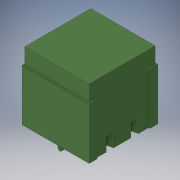
# Autodesk Inventor part: M211LW01-body
Saved by Autodesk Inventor 2019 (Build 230136000, 136)
## iProperties
Created: 2022-08-22
Part Number: M211LW01-body
Material: Generic
Catalog Web Link: www.cadenas.de
Description: Series M2100 - LED Tipped Actuators - body-
Vendor: NKKSWITCHES
Document SubType Name: Modeling
Designer: psAdmin
Manufacturer: NKKSWITCHES
Mass: 2.03481 g
Surface Area: 10.5273 cm^2
Volume: 2.03481 cm^3
Density: 1 g/cm^3
Appearance: PSOLRGB-79-119-66
Category: PARTsolutions
Company: NKKSWITCHES
Title: M211LW01-body
Author: Cadenas PARTsolutions
PSOL_IDENT_0: {$CADENAS_DATA/23d-libs/nkkswitches/toggle/m2100/parts/m2100_body.prj},219 {VTYP=3D},{NB=M211LW01-bo
PSOL_IDENT_1: dy},{LINA=M211LW01-body},{NN=Series M2100 - LED Tipped Actuators - body},{DATE=02.08.2022 07:27:12},
PSOL_IDENT_2: {GEOMDATE=10.04.2009 08:21:00},{VERSION=},{LINEID=10},{WBVAR=PLS,LCAT,CMRT,TMT},{WBNUMERIC=}  {NB=M2
PSOL_IDENT_3: 11LW01-body},{LINA=M211LW01-body},{KT=DUMMY},{PN=M211LW01},{SRS=M21},{PLS=1},{LCAT=L},{LCAT1= 'L','L
PSOL_IDENT_4: - Isolated (Toggle)','T','T - Synchronous (Toggle)','R','R - Isolated (Rocker)','N','N - Synchronou
PSOL_IDENT_5: s (Rocker)','P','P - Isolated (Paddle)','J','J - Synchronous (Paddle)' },{CMRT=W},{TMT=01},{TMT1= '0
PSOL_IDENT_6: 1','01 - Solder Lug with Threaded Bushing','02','02 - Quick Connect with Threaded Bushing','03','03
PSOL_IDENT_7: - Straight PC with Threaded Bushing' }
NB: M211LW01-body
NN: Series M2100 - LED Tipped Actuators - body
NBSYN: $PN.-body
LINA: M211LW01-body
CATALOG: NKK Switches
PN: M211LW01
SRS: M21
PLS: 1 - SPDT
LCAT: L - Isolated (Toggle)
CMRT: W - Silver; Rated 6A @ 125V AC
TMT: 01 - Solder Lug with Threaded Bushing
SUPPLIER: NKKSWITCHES
ARTICLENO: M211LW01-body
BOMINFO: M211LW01-body
CREATOR: CADENAS GmbH
Autodesk Inventor part; units mm, degrees
sketch "Sketch_1" plane through (0, 0, 0) normal (1, 0, 0) x (0, 1, 0)
  line L0 (12.8016, 6.5024) -> (0, 6.5024)
  line L1 (0, 6.5024) -> (0, -6.5024)
  line L2 (0, -6.5024) -> (12.8016, -6.5024)
  line L3 (12.8016, -6.5024) -> (12.8016, 6.5024)
  constraints: 8 end point
extrude "Extrusion1" add sketch "Sketch_1" along normal mid plane 12.7
sketch "Sketch_5" plane through (6.35, 0, 0) normal (1, 0, 0) x (0, 0, -1)
  line L0 (-6.5024, 9.7536) -> (-5.4864, 9.7536)
  arc A0 (-4.9784, 9.2456) -> (-5.4864, 9.7536) centre (-5.4864, 9.2456) ccw
  line L1 (-4.9784, 9.2456) -> (-4.9784, 0)
  line L2 (-4.9784, 0) -> (4.9784, 0)
  line L3 (4.9784, 0) -> (4.9784, 9.2456)
  arc A1 (5.4864, 9.7536) -> (4.9784, 9.2456) centre (5.4864, 9.2456) ccw
  line L4 (5.4864, 9.7536) -> (6.5024, 9.7536)
  line L5 (6.5024, 9.7536) -> (6.5024, 13.0556)
  line L6 (6.5024, 13.0556) -> (-6.5024, 13.0556)
  line L7 (-6.5024, 13.0556) -> (-6.5024, 9.7536)
  constraints: 16 end point, 4 point on circle, 2 centre point
extrude "Extrusion2" cut sketch "Sketch_5" against normal blind 0.254
sketch "Sketch_6" plane through (-6.35, 0, 0) normal (1, 0, 0) x (0, 0, -1)
  line L0 (-6.5024, 9.7536) -> (-5.4864, 9.7536)
  arc A0 (-4.9784, 9.2456) -> (-5.4864, 9.7536) centre (-5.4864, 9.2456) ccw
  line L1 (-4.9784, 9.2456) -> (-4.9784, 0)
  line L2 (-4.9784, 0) -> (4.9784, 0)
  line L3 (4.9784, 0) -> (4.9784, 9.2456)
  arc A1 (5.4864, 9.7536) -> (4.9784, 9.2456) centre (5.4864, 9.2456) ccw
  line L4 (5.4864, 9.7536) -> (6.5024, 9.7536)
  line L5 (6.5024, 9.7536) -> (6.5024, 13.0556)
  line L6 (6.5024, 13.0556) -> (-6.5024, 13.0556)
  line L7 (-6.5024, 13.0556) -> (-6.5024, 9.7536)
  constraints: 16 end point, 4 point on circle, 2 centre point
extrude "Extrusion3" cut sketch "Sketch_6" along normal blind 0.254
sketch "Sketch_7" plane through (0, 0, -6.5024) normal (0, 0, 1) x (1, 0, 0)
  line L0 (-6.35, 9.7536) -> (6.35, 9.7536)
  line L1 (6.35, 9.7536) -> (6.35, 13.0556)
  line L2 (6.35, 13.0556) -> (-6.35, 13.0556)
  line L3 (-6.35, 13.0556) -> (-6.35, 9.7536)
  constraints: 8 end point
extrude "Extrusion4" cut sketch "Sketch_7" along normal blind 0.254
sketch "Sketch_8" plane through (0, 0, 6.5024) normal (0, 0, 1) x (1, 0, 0)
  line L0 (-6.35, 9.7536) -> (6.35, 9.7536)
  line L1 (6.35, 9.7536) -> (6.35, 13.0556)
  line L2 (6.35, 13.0556) -> (-6.35, 13.0556)
  line L3 (-6.35, 13.0556) -> (-6.35, 9.7536)
  constraints: 8 end point
extrude "Extrusion5" cut sketch "Sketch_8" against normal blind 0.254
sketch "Sketch_9" plane through (0, 0, 0) normal (0, 1, 0) x (-1, 0, 0)
  line L0 (8.128, 8.2804) -> (-8.128, 8.2804)
  line L1 (-8.128, 8.2804) -> (-8.128, -8.2804)
  line L2 (-8.128, -8.2804) -> (8.128, -8.2804)
  line L3 (8.128, -8.2804) -> (8.128, 8.2804)
  line L4 (6.35, -1.5875) -> (6.35, 1.5875)
  line L5 (6.35, 1.5875) -> (5.08, 1.8415)
  line L6 (5.08, 1.8415) -> (5.08, 2.8575)
  line L7 (5.08, 2.8575) -> (6.35, 3.1115)
  line L8 (6.35, 3.1115) -> (6.35, 6.5024)
  line L9 (6.35, 6.5024) -> (-6.35, 6.5024)
  line L10 (-6.35, 6.5024) -> (-6.35, 3.1115)
  line L11 (-6.35, 3.1115) -> (-5.08, 2.8575)
  line L12 (-5.08, 2.8575) -> (-5.08, 1.8415)
  line L13 (-5.08, 1.8415) -> (-6.35, 1.5875)
  line L14 (-6.35, 1.5875) -> (-6.35, -1.5875)
  line L15 (-6.35, -1.5875) -> (-5.08, -1.8415)
  line L16 (-5.08, -1.8415) -> (-5.08, -2.8575)
  line L17 (-5.08, -2.8575) -> (-6.35, -3.1115)
  line L18 (-6.35, -3.1115) -> (-6.35, -6.5024)
  line L19 (-6.35, -6.5024) -> (6.35, -6.5024)
  line L20 (6.35, -6.5024) -> (6.35, -3.1115)
  line L21 (6.35, -3.1115) -> (5.08, -2.8575)
  line L22 (5.08, -2.8575) -> (5.08, -1.8415)
  line L23 (5.08, -1.8415) -> (6.35, -1.5875)
  constraints: 48 end point
extrude "Extrusion6" cut sketch "Sketch_9" along normal blind 2.54
sketch "Sketch_10" plane through (0, 0, 0) normal (0, 0, 1) x (1, 0, 0)
  line L0 (-0.381, 0) -> (-0.381, -1.1684)
  arc A0 (-0.381, -1.1684) -> (0.381, -1.1684) centre (0, -1.1684) ccw
  line L1 (0.381, -1.1684) -> (0.381, 0)
  line L2 (0.381, 0) -> (-0.381, 0)
  constraints: 6 end point, 2 point on circle, 1 centre point
extrude "Extrusion7" add sketch "Sketch_10" along normal mid plane 11.43
sketch "Sketch_11" plane through (0, 0, 0) normal (1, 0, 0) x (0, 1, 0)
  arc A0 (-0.381, 2.7305) -> (-0.381, 1.9685) centre (-0.381, 2.3495) ccw
  line L0 (-0.381, 1.9685) -> (0, 1.9685)
  line L1 (0, 1.9685) -> (0, -1.9685)
  line L2 (0, -1.9685) -> (-0.381, -1.9685)
  arc A1 (-0.381, -1.9685) -> (-0.381, -2.7305) centre (-0.381, -2.3495) ccw
  line L3 (-0.381, -2.7305) -> (0.508, -2.7305)
  line L4 (0.508, -2.7305) -> (0.508, 2.7305)
  line L5 (0.508, 2.7305) -> (-0.381, 2.7305)
  constraints: 12 end point, 4 point on circle, 2 centre point
extrude "Extrusion8" add sketch "Sketch_11" along normal mid plane 9.144
ref_plane "body_to_body_c_XY" through (0, 12.8016, 0) normal (0, -1, 0) x (1, 0, 0)
ref_plane "body_to_body_c_YZ" through (0, 12.8016, 0) normal (1, 0, 0) x (0, 0, 1)
ref_plane "body_to_body_c_ZX" through (0, 12.8016, 0) normal (0, 0, 1) x (0, -1, 0)
ref_plane "body_to_dummy_XY" through (0, 0, 0) normal (0, -1, 0) x (1, 0, 0)
ref_plane "body_to_dummy_YZ" through (0, 0, 0) normal (1, 0, 0) x (0, 0, 1)
ref_plane "body_to_dummy_ZX" through (0, 0, 0) normal (0, 0, 1) x (0, -1, 0)
ref_plane "body_to_terminal_XY" through (0, 0, 0) normal (0, -1, 0) x (1, 0, 0)
ref_plane "body_to_terminal_YZ" through (0, 0, 0) normal (1, 0, 0) x (0, 0, 1)
ref_plane "body_to_terminal_ZX" through (0, 0, 0) normal (0, 0, 1) x (0, -1, 0)
body "Solid1"
